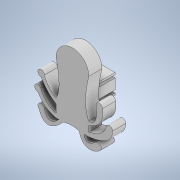
# Autodesk Inventor part: octopus_on_belt
Saved by Autodesk Inventor 2020 (Build 240168000, 168)
## iProperties
Created: 2021-03-06
Part Number: octopus_on_belt
Material: Generic
Document SubType Name: Modeling
Designer: Harry
Density: 1 g/cm^3
Appearance: Default
Author: Harry
Autodesk Inventor part; units mm, degrees
ref_plane "YZ Plane" through (0, 0, 0) normal (1, 0, 0) x (0, 1, 0)
ref_plane "XZ Plane" through (0, 0, 0) normal (0, 1, 0) x (-1, 0, 0)
ref_plane "XY Plane" through (0, 0, 0) normal (0, 0, 1) x (1, 0, 0)
sketch "Sketch2" plane through (0, 0, 0) normal (0, 0, 1) x (1, 0, 0)
  line L0 (-12.5, -16.8475) -> (-12.5, -10.7194)
  line L1 (12.5, -12.5194) -> (12.5, -16.8475)
  line L2 (12.5, -20) -> (-12.5, 20) construction
  line L3 (-12.5, -20) -> (12.5, 20) construction
  arc A0 (12.5, 20) -> (-12.5, 20) centre (0, 20) ccw
  arc A1 (-23.9938, -6.3332) -> (-26.3611, -9.6367) centre (-26.3611, -7.1367) ccw
  arc A2 (-21.3611, 3.8099) -> (-23.8611, 1.3099) centre (-23.8611, 3.8099) ccw
  arc A3 (-21.3611, -18.5591) -> (-25.4614, -20.4798) centre (-23.8611, -18.5591) ccw
  arc A4 (22.9392, 3.8099) -> (18.0516, 3.0686) centre (20.4392, 3.8099) ccw
  arc A5 (30.6335, -7.1367) -> (25.6339, -7.1814) centre (28.1335, -7.1367) ccw
  arc A6 (21.1908, -24.646) -> (17.9392, -20.8491) centre (19.6037, -22.7144) ccw
  spline S0 degree 2 poles (-23.8611, 1.3099) (-19.0526, -6.9708) (-12.5, -10.7194) knots 0 0 0 1 1 1
  spline S1 degree 2 poles (-21.3611, 3.8099) (-18.5864, -3.6522) (-12.5, -6.6832) knots 0 0 0 1 1 1
  spline S2 degree 2 poles (-26.3611, -9.6367) (-21.4971, -18.1116) (-12.5, -20) knots 0 0 0 1 1 1
  spline S3 degree 2 poles (-24.0407, -6.2062) (-21.0395, -14.4004) (-12.5, -16.8475) knots 0 0 0 1 1 1
  spline S4 degree 2 poles (-21.3611, -18.5591) (-18.1547, -28.3248) (-10.356, -20) knots 0 0 0 1 1 1
  spline S5 degree 2 poles (-25.4614, -20.4798) (-20.4927, -34.7918) (-6.9898, -20) knots 0 0 0 1 1 1
  spline S6 degree 2 poles (17.9392, 3.8099) (20.0689, -9.5172) (12.5, -9.6367) knots 0 0 0 1 1 1
  spline S7 degree 2 poles (22.9392, 3.8099) (24.5184, -8.2792) (12.5, -12.5194) knots 0 0 0 1 1 1
  spline S8 degree 2 poles (25.8131, -6.2062) (24.8315, -13.7331) (12.5, -16.8475) knots 0 0 0 1 1 1
  spline S9 degree 2 poles (30.6335, -7.1367) (30.4955, -17.6904) (12.5, -20) knots 0 0 0 1 1 1
  spline S10 degree 2 poles (9.1202, -20) (9.7376, -27.3779) (17.9392, -20.8491) knots 0 0 0 1 1 1
  spline S11 degree 3 poles (21.1908, -24.646) (15.8936, -29.7076) (6.4999, -29.4415) (5.3692, -20) knots 0 0 0 0 1 1 1 1
  spline S12 degree 2 poles (12.5, 20) (7.4894, -0.1647) (12.5, -9.6367) knots 0 0 0 1 1 1
  spline S13 degree 2 poles (-12.5, 20) (-7.9354, -0.2578) (-12.5, -6.6832) knots 0 0 0 1 1 1
  line L4 (12.5, -20) -> (9.1202, -20)
  line L5 (-10.356, -20) -> (-12.5, -20)
  spline S14 degree 2 poles (-6.9898, -20) (0.0212, -17.9924) (5.3692, -20) knots 0 0 0 1 1 1
  point P0 (0, 0)
  point P1 (-18.2659, -6.203)
  point P2 (-17.5697, -2.7642)
  point P3 (-20.3482, -16.5508)
  point P4 (-19.6835, -12.9372)
  point P5 (-17.232, -23.7647)
  point P6 (-19.3511, -27.4539)
  point P7 (17.0045, -7.4262)
  point P8 (21.1905, -6.2037)
  point P9 (22.9403, -11.7957)
  point P10 (27.4494, -14.4708)
  point P11 (11.0482, -23.7717)
  point P12 (14.8952, -27.8035)
  point P13 (9.1239, -26.7454)
  point P14 (10.0714, -0.0017)
  point P15 (-10.3694, -0.0099)
  point P16 (0, -19.0003)
  dimension "d6" = 40
  dimension "d7" = 25
  dimension "d8" = 5
  dimension "d9" = 5
  dimension "d10" = 5
  dimension "d11" = 5
  dimension "d12" = 5
  dimension "d13" = 5
  constraints: 17 point on circle, 12 end point, 7 centre point, 2 horizontal, 2 perpendicular, 1 parallel, 68 other
  measures "d6" distance of L3.start L2.end
  measures "d7" distance of L2.start L3.start
  measures "d8" diameter of A1
  measures "d9" diameter of A2
  measures "d10" diameter of A3
  measures "d11" diameter of A4
  measures "d12" diameter of A5
  measures "d13" diameter of A6
extrude "Extrusion1" add sketch "Sketch2" along normal blind 10 contours L0 S0 A2 S1 S13 A0 S12 S6 A4 S7 L1 S8 A5 S9 L4 S10 A6 S11 S14 S5 A3 S4 L5 S2 A1 S3
sketch "Sketch3" plane through (0, 0, 0) normal (0, 0, -1) x (-1, 0, 0)
  line L0 (7.5, -7.5) -> (-7.5, -7.5)
  line L1 (-7.5, -7.5) -> (-7.5, 7.5)
  line L2 (-7.5, 7.5) -> (7.5, 7.5)
  line L3 (7.5, 7.5) -> (7.5, -7.5)
  line L4 (7.5, -7.5) -> (-7.5, 7.5) construction
  line L5 (-7.5, -7.5) -> (7.5, 7.5) construction
  point P0 (0, 0)
  dimension "d16" = 15
  dimension "d17" = 15
  constraints: 12 end point, 2 midpoint, 2 parallel, 1 horizontal, 1 perpendicular
  measures "d16" distance of L1.end L2.end
  measures "d17" distance of L0.end L1.end
extrude "Extrusion2" add sketch "Sketch3" along normal blind 15
sketch "Sketch4" plane through (0, 0, -15) normal (0, 0, -1) x (-1, 0, 0)
  line L0 (0, 0) -> (0, 5) construction
  line L1 (0, 0) -> (0, -5) construction
  line L2 (7.5, 4) -> (-7.5, 4)
  line L3 (-7.5, 4) -> (-7.5, 6)
  line L4 (-7.5, 6) -> (7.5, 6)
  line L5 (7.5, 6) -> (7.5, 4)
  line L6 (7.5, 4) -> (-7.5, 6) construction
  line L7 (-7.5, 4) -> (7.5, 6) construction
  line L8 (7.5, -6) -> (-7.5, -6)
  line L9 (-7.5, -6) -> (-7.5, -4)
  line L10 (-7.5, -4) -> (7.5, -4)
  line L11 (7.5, -4) -> (7.5, -6)
  line L12 (7.5, -6) -> (-7.5, -4) construction
  line L13 (-7.5, -6) -> (7.5, -4) construction
  dimension "d20" = 5
  dimension "d21" = 5
  dimension "d22" = 15
  dimension "d23" = 2
  dimension "d24" = 15
  dimension "d25" = 2
  constraints: 28 end point, 4 midpoint, 4 parallel, 2 horizontal, 2 perpendicular, 2 vertical
  measures "d20" distance of L0.start L0.end
  measures "d21" distance of L0.start L1.end
  measures "d22" distance of L3.end L4.end
  measures "d23" distance of L2.end L3.end
  measures "d24" distance of L9.end L10.end
  measures "d25" distance of L8.end L9.end
extrude "Extrusion3" cut sketch "Sketch4" against normal blind 15
body "Solid1"
